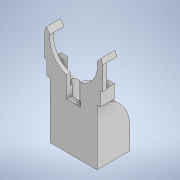
# Autodesk Inventor part: MouseCover_v2
Saved by Autodesk Inventor 2021 (Build 250183000, 183)
## iProperties
Created: 2021-07-17
Part Number: MouseCover_v2
Material: Generic
Document SubType Name: Modeling
Designer: scanimage
Density: 1 g/cm^3
Appearance: Default
Author: scanimage
Autodesk Inventor part; units mm, degrees
ref_plane "YZ Plane" through (0, 0, 0) normal (1, 0, 0) x (0, 1, 0)
ref_plane "XZ Plane" through (0, 0, 0) normal (0, 1, 0) x (-1, 0, 0)
ref_plane "XY Plane" through (0, 0, 0) normal (0, 0, 1) x (1, 0, 0)
sketch "Sketch1" plane through (0, 0, 0) normal (0, 0, 1) x (1, 0, 0)
  line L0 (-43.561, 0) -> (43.561, 0) projected
  line L1 (0, -8) -> (0, 48) projected
  line L2 (31.115, 40) -> (31.115, 0)
  line L3 (-31.115, 40) -> (-31.115, 0)
  line L4 (-31.115, 0) -> (31.115, 0)
  line L5 (-31.115, 40) -> (-25.115, 40)
  line L6 (31.115, 40) -> (25.115, 40)
  arc A0 (-25.115, 40) -> (25.115, 40) centre (0, 36) ccw
  line L7 (-31.115, 0) -> (31.115, 0)
  line L8 (-31.115, 0) -> (31.115, 0)
  point P0 (0, 0)
  dimension "d0" = 62.23
  dimension "d1" = 40
  dimension "d2" = 6
  dimension "d3" = 6
  dimension "d4" = 4
  dimension "d57" = 50.23
  dimension "d60" = 0
  constraints: 14 end point, 3 collinear, 2 horizontal, 2 perpendicular, 2 point on circle, 2 point on line, 1 centre point
  measures "d0" distance of L3.start L2.start
  measures "d1" distance of L3.start L3.end
  measures "d2" distance of L3.start L5.end
  measures "d3" distance of L2.start L6.end
  measures "d4" vertical distance of A0.centre L5.end
  measures "d57" distance of L5.end L6.end
  measures "d60" distance from line of L1 A0.centre
extrude "Extrusion1" add sketch "Sketch1" against normal blind 4
sketch "Sketch3" plane through (0, 0, 0) normal (0, 0, 1) x (1, 0, 0)
  line L0 (0, -72) -> (0, 12) projected
  line L1 (-25, 0) -> (25, 0)
  line L2 (-25, 0) -> (-25, -60)
  line L3 (25, 0) -> (25, -60)
  line L4 (-25, -60) -> (25, -60)
  point P0 (0, 0)
  dimension "d15" = 60
  dimension "d16" = 50
  dimension "d17" = 25
  constraints: 8 end point, 2 vertical, 1 horizontal
  measures "d15" distance of L1.start L2.end
  measures "d16" distance of L1.start L1.end
  measures "d17" distance of L1.end point (0, 0)
extrude "Extrusion3" add sketch "Sketch3" against normal blind 35
sketch "Sketch5" plane through (-25, 0, -4) normal (0, 1, 0) x (1, 0, 0)
  line L0 (-18.561, -4) -> (68.561, -4) projected
  line L1 (25, 38) -> (25, -11) projected
  line L2 (0, 31) -> (50, 31) projected
  arc A0 (10, 31) -> (40, 31) centre (25, 19.75) ccw
  point P0 (25, -4)
  dimension "d20" = 30
  dimension "d21" = 15
  dimension "d22" = 15
  constraints: 2 point on circle, 2 point on line, 1 centre point
  measures "d21" distance from line of L1 A0.start
  measures "d22" distance from line of A0.end L1
extrude "Extrusion4" cut sketch "Sketch5" against normal blind 75
chamfer "Chamfer2" distance 8.89 angle 45 2 edges at (-15, -30, -35) (15, -30, -35)
fillet "Fillet1" radius 6.35 2 edges at (18.4959, -30, -26.8262) (-18.4959, -30, -26.8262)
fillet "Fillet2" radius 38.1 2 edges at (24.445, 0, -35) (-24.445, 0, -35)
sketch "Sketch6" plane through (0, 0, 0) normal (0, 0, 1) x (1, 0, 0)
  line L0 (-43.561, 0) -> (43.561, 0) projected
  line L1 (0, -81) -> (0, 66) projected
  line L2 (-31.115, 0) -> (-31.115, 40) projected
  line L3 (-31.115, 40) -> (-29.115, 45)
  line L4 (-31.115, 40) -> (-25.115, 40) projected
  line L5 (-29.115, 45) -> (-25.115, 40)
  line L6 (25.115, 40) -> (31.115, 40) projected
  line L7 (31.115, 40) -> (29.115, 45)
  line L8 (29.115, 45) -> (25.115, 40)
  line L9 (31.115, 0) -> (31.115, 40) projected
  point P0 (0, 0)
  dimension "d33" = 5
  dimension "d34" = 2
  dimension "d37" = 5
  dimension "d38" = 2
  constraints: 8 end point
  measures "d33" distance from line of L4 L3.end
  measures "d34" horizontal distance of L2.end L3.end
  measures "d37" distance from line of L7.end L6
  measures "d38" distance from line of L9 L7.end
extrude "Extrusion5" add sketch "Sketch6" against normal blind 15
sketch "Sketch7" plane through (0, 0, 0) normal (0, 0, 1) x (1, 0, 0)
  line L0 (-43.561, 0) -> (43.561, 0) projected
  line L1 (0, -81) -> (0, 66) projected
  line L2 (-31.115, 0) -> (-31.115, 40) projected
  line L3 (-25, 0) -> (-25, -60) projected
  line L4 (31.115, 40) -> (31.115, 0) projected
  line L5 (25, 0) -> (-25, 0) projected
  line L6 (-30.48, 0) -> (-21.59, 0)
  line L7 (-21.59, 0) -> (-21.59, 14.092)
  line L8 (-21.59, 14.092) -> (-30.48, 14.092)
  line L9 (-30.48, 14.092) -> (-30.48, 0)
  line L10 (21.59, 0) -> (21.59, 14.092)
  line L11 (21.59, 14.092) -> (30.48, 14.092)
  line L12 (30.48, 14.092) -> (30.48, 0)
  point P0 (0, 0)
  dimension "d58" = 8.89
  dimension "d59" = 21.59
  constraints: 14 end point, 4 symmetric about line, 2 parallel, 1 horizontal, 1 perpendicular, 1 point on line
  measures "d58" distance between parallel lines of L7 L9
  measures "d59" distance between parallel lines of L1 L7
extrude "Extrusion6" add sketch "Sketch7" against normal blind 15
sketch "Sketch8" plane through (0, 0, 0) normal (0, 0, 1) x (1, 0, 0)
  line L0 (-43.561, 0) -> (43.561, 0) projected
  line L1 (0, -81) -> (0, 66) projected
  line L2 (0, -10.6734) -> (7.62, -10.6734)
  line L3 (7.62, -10.6734) -> (7.62, 14.7266)
  line L4 (7.62, 14.7266) -> (0, 14.7266)
  line L5 (-7.62, 14.7266) -> (-7.62, -10.6734)
  line L6 (-7.62, -10.6734) -> (0, -10.6734)
  line L7 (0, 14.7266) -> (-7.62, 14.7266)
  point P0 (0, 0)
  dimension "d46" = 25.4
  dimension "d47" = 7.62
  dimension "d48" = 7.62
  constraints: 12 end point, 5 perpendicular, 4 point on line, 1 parallel
  measures "d46" distance of L2.end L3.end
  measures "d47" distance of L2.start L2.end
  measures "d48" distance of L4.end L5.start
extrude "Extrusion7" cut sketch "Sketch8" against normal blind 25.4
sketch "Sketch9" plane through (31.115, 0, 0) normal (1, 0, 0) x (0, 0, -1)
  line L0 (0, 15.24) -> (15, 15.24)
  line L1 (15, 15.24) -> (15, 0)
  line L2 (15, 0) -> (0, 0)
  line L3 (0, 0) -> (0, 15.24)
  point P0 (0, 0)
  dimension "d53" = 15.24
  constraints: 8 end point, 2 parallel, 1 horizontal, 1 perpendicular
  measures "d53" distance between parallel lines of L2 L0
extrude "Extrusion8" cut sketch "Sketch9" against normal blind 2.54
sketch "Sketch10" plane through (-31.115, 0, 0) normal (-1, 0, 0) x (0, 0, 1)
  line L0 (-15, 14.092) -> (-15, 0) projected
  line L1 (0, 0) -> (0, 15.24) projected
  line L2 (-15, 15.24) -> (0, 15.24)
  line L3 (0, 15.24) -> (0, 0)
  line L4 (0, 0) -> (-15, 0)
  line L5 (-15, 0) -> (-15, 15.24)
  point P0 (-15, 13.97)
  point P1 (0, 15.24)
  point P2 (-15, 0)
  point P3 (-15, 0)
  point P4 (0, 15.24)
  dimension "d54" = 15.24
  constraints: 8 end point, 2 parallel, 1 horizontal, 1 perpendicular, 1 point on line
  measures "d54" distance between parallel lines of L4 L2
extrude "Extrusion9" cut sketch "Sketch10" against normal blind 2.54
equation "\"d3\" = d2"
equation "\"d57\" = d0 - 2 * d2"
equation "\"d22\" = d21"
equation "\"d37\" = d33"
equation "\"d38\" = d34"
equation "\"d48\" = d47"
body "Solid1"
